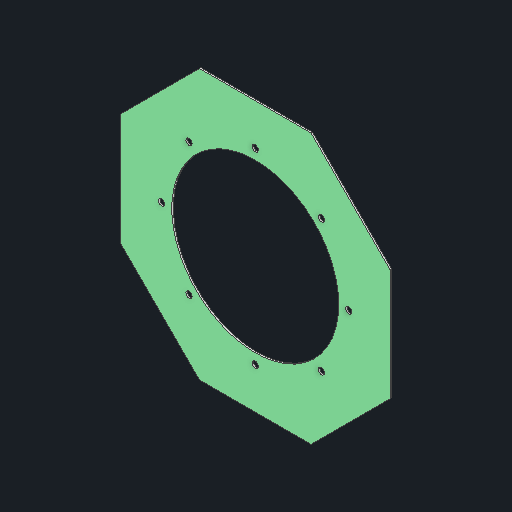
# Autodesk Inventor part: DMF 01 22 Барабан торец КОРМА v2.1
Saved by Autodesk Inventor 2026.2 (Build 302298010, 298A)
## iProperties
Created: 2024-04-28
Part Number: DMF 01 22 Барабан торец КОРМА v2.1
Material: Generic
Document SubType Name: Sheet Metal
Designer: pokla
Density: 1 g/cm^3
Appearance: Default
Sheet Metal Rule: Default
Flat Pattern Width: 53 cm
Flat Pattern Length: 53 cm
Flat Pattern Area: 2809 cm^2
Sheet Metal Width: 530,000 mm
Sheet Metal Length: 530,000 mm
Sheet Metal Area: 280900,000 mm^2
Stock Number: Барабан_Торец_Корма
Author: pokla
Autodesk Inventor part; units mm, degrees
ref_plane "YZ Plane" through (0, 0, 0) normal (1, 0, 0) x (0, 1, 0)
ref_plane "XZ Plane" through (0, 0, 0) normal (0, 1, 0) x (-1, 0, 0)
ref_plane "XY Plane" through (0, 0, 0) normal (0, 0, 1) x (1, 0, 0)
sketch "Sketch2" plane through (0, 0, 0) normal (0, 0, 1) x (1, 0, 0)
  line L0 (-265, 109.7666) -> (-109.7666, 265)
  line L1 (-109.7666, 265) -> (109.7666, 265)
  line L2 (109.7666, 265) -> (265, 109.7666)
  line L3 (265, 109.7666) -> (265, -109.7666)
  line L4 (265, -109.7666) -> (109.7666, -265)
  line L5 (109.7666, -265) -> (-109.7666, -265)
  line L6 (-109.7666, -265) -> (-265, -109.7666)
  line L7 (-265, -109.7666) -> (-265, 109.7666)
  circle A0 centre (0, 0) radius 164
  point P0 (0, 265)
  dimension "d23" = 530
  dimension "d26" = 328
  measures "d23" distance between parallel lines of L6 L2
  measures "d26" diameter of A0
extrude "Plate1" add sketch "Sketch2" against normal blind 3
sketch "Sketch4" plane through (0, 0, 0) normal (0, 0, 1) x (1, 0, 0)
  circle A0 centre (0, 184) radius 6.25
  circle A1 centre (0, 0) radius 164 projected
  dimension "d16" = 12.5
  dimension "d17" = 184
  constraints: 1 centre point, 1 vertical alignment
  measures "d16" diameter of A0
  measures "d17" distance of point (0, 0) A0.centre
extrude "Extrusion1" cut sketch "Sketch4" against normal up to surface (3 mm away) contours A0
pattern_circular "Circular Pattern1" count 8 over 360 about axis through (0, 0, -10) along (0, 0, 1) of "Extrusion1"
equation "\"d23\" = Барабан_размер_по_плоскостям"
equation "\"d15\" = Thickness"
equation "\"BendRadius\" = Thickness"
equation "\"BendReliefWidth\" = Thickness"
equation "\"BendReliefDepth\" = 0.5 * Thickness"
equation "\"CornerReliefSize\" = 4 * Thickness"
equation "\"MinimumRemnant\" = 2 * Thickness"
equation "\"TransitionRadius\" = BendRadius"
equation "\"JacobiRadiusSize\" = BendRadius"
equation "\"GapSize\" = Thickness"
equation "\"Барабан_размер_по_плоскостям\" = 530"
equation "\"Thickness\" = 3"
body "Solid1"
